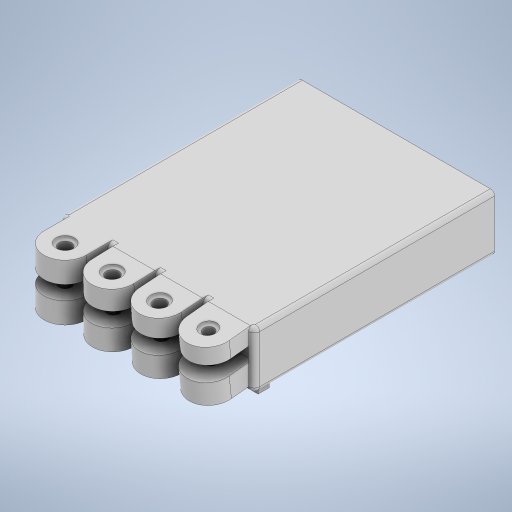
# Autodesk Inventor part: baze
Saved by Autodesk Inventor 2024 (Build 280153000, 153)
## iProperties
Created: 2023-12-07
Part Number: baze
Material: Типовые
Document SubType Name: Modeling
Designer: stefa
Density: 1 g/cm^3
Appearance: По умолчанию
Author: stefa
Autodesk Inventor part; units mm, degrees
ref_plane "YZ Plane" through (0, 0, 0) normal (1, 0, 0) x (0, 1, 0)
ref_plane "XZ Plane" through (0, 0, 0) normal (0, 1, 0) x (-1, 0, 0)
ref_plane "XY Plane" through (0, 0, 0) normal (0, 0, 1) x (1, 0, 0)
sketch "Эскиз1" plane through (0, 0, 0) normal (1, 0, 0) x (0, 1, 0)
  line L0 (0, 0) -> (20, 0)
  line L1 (20, 0) -> (20, -100)
  line L2 (20, -100) -> (0, -100)
  line L3 (0, -100) -> (0, 0)
  line L4 (12.5, 0) -> (12.5, -15)
  line L5 (12.5, -15) -> (7.5, -15)
  line L6 (7.5, -15) -> (7.5, 0)
  line L7 (7.5, 0) -> (12.5, 0)
  dimension "d0" = 20
  dimension "d1" = 100
  dimension "d2" = 15
  dimension "d3" = 5
  dimension "d4" = 7.5
  dimension "d5" = 7.5
  constraints: 16 end point, 4 parallel, 3 perpendicular, 1 horizontal, 1 point on line
  measures "d0" distance of L0.start L0.end
  measures "d1" distance of L0.end L1.end
  measures "d2" distance of L5.end L6.end
  measures "d3" distance of L4.end L5.end
  measures "d4" distance between parallel lines of L1 L4
  measures "d5" distance between parallel lines of L3 L6
extrude "Выдавливание1" add sketch "Эскиз1" along normal blind 15 contours L0 L6 L5 L4 L1 L2 L3
sketch "Эскиз2" plane through (15, 0, 0) normal (1, 0, 0) x (0, 0, -1)
  line L0 (0, 0) -> (100, 0) projected
  line L1 (100, 20) -> (0, 20) projected
  line L2 (100, 0) -> (15, 0)
  line L3 (15, 0) -> (15, 20)
  line L4 (15, 20) -> (100, 20)
  line L5 (100, 20) -> (100, 0)
  dimension "d8" = 85
  constraints: 8 end point, 2 parallel, 1 horizontal, 1 perpendicular, 1 point on line
  measures "d8" distance of L3.end L4.end
extrude "Выдавливание2" add sketch "Эскиз2" along normal blind 2
sketch "Эскиз3" plane through (17, 0, 0) normal (1, 0, 0) x (0, 0, -1)
  line L0 (100, 0) -> (100, 20)
  line L1 (0, 0) -> (100, 0)
  line L2 (100, 0) -> (100, 20)
  line L3 (100, 20) -> (0, 20)
  line L4 (0, 20) -> (0, 0)
  line L5 (0, 12.503049) -> (15, 13.02686)
  line L6 (15, 13.02686) -> (15.174604, 8.02686)
  line L7 (15.174604, 8.02686) -> (0, 7.496951)
  line L8 (0, 12.5) -> (15, 12.5)
  line L9 (0, 19.476188) -> (15, 20)
  line L10 (0, 0) -> (15, 0.523812)
  line L11 (15, 20) -> (15, 0)
  line L12 (15, 20) -> (15, 13.02686)
  line L13 (15.174604, 8.02686) -> (15, 0.523812)
  line L14 (15, 0) -> (15, 0.523812)
  line L15 (0, 19.476188) -> (0.243211, 12.511542)
  line L16 (0, 7.496951) -> (0.26148, 0.009131)
  dimension "d11" = 88
  dimension "d12" = 90
  dimension "d13" = 88
  dimension "d14" = 15
  dimension "d15" = 5
  dimension "d16" = 7.49695
  dimension "d17" = 7.49695
  dimension "d18" = 2
  dimension "d35" = 2
  dimension "d36" = 178
  dimension "d50" = 2
  dimension "d51" = 2
  constraints: 28 end point, 7 point on line, 2 parallel, 2 perpendicular, 1 collinear, 1 horizontal
  measures "d11" angle of L5 L4
  measures "d12" angle of L6 L7
  measures "d13" angle of L4 L7
  measures "d14" horizontal distance of L5.start L5.end
  measures "d15" vertical distance of L5.end L6.end
  measures "d16" distance of L3.end L5.start
  measures "d17" distance of L1.start L7.end
  measures "d18" angle of L8 L5
  measures "d35" angle of L3 L9
  measures "d36" angle of L1 L10
  measures "d50" angle of L15 L4
  measures "d51" angle of L16 L4
extrude "Выдавливание3" add sketch "Эскиз3" along normal blind 15 contours L1 L11 L13 L6 L3 L0 | L11 L5 L15 L9 | L10 L16 L7 L11 | L11 L7 L13
sketch "Эскиз4" plane through (32, 0, 0) normal (1, 0, 0) x (0, 0, -1)
  line L0 (15, 0) -> (15, 7.5) projected
  line L1 (100, 20) -> (15, 20) projected
  line L2 (15, 0) -> (100, 0)
  line L3 (100, 0) -> (100, 20)
  line L4 (100, 20) -> (15, 20)
  line L5 (15, 20) -> (15, 0)
  point P0 (0, 0)
  point P1 (0, 20)
  point P2 (15, 20)
  constraints: 8 end point, 2 parallel, 1 horizontal, 1 perpendicular
extrude "Выдавливание4" add sketch "Эскиз4" along normal blind 2
sketch "Эскиз5" plane through (34, 0, 0) normal (1, 0, 0) x (0, 0, -1)
  line L0 (15, 20) -> (0, 20)
  line L1 (100, 0) -> (100, 20)
  line L2 (0, 20) -> (100, 20)
  line L3 (100, 20) -> (100, 0)
  line L4 (100, 0) -> (0, 0)
  line L5 (0, 0) -> (0, 20)
  line L6 (0, 12.5) -> (15, 13.548902)
  line L7 (15, 13.548902) -> (15.347933, 8.573232)
  line L8 (15.347933, 8.573232) -> (0, 7.5)
  line L9 (15, 12.5) -> (15, 20)
  line L10 (0, 18.951098) -> (15, 20)
  line L11 (0, 0) -> (15, 1.048902)
  line L12 (15, 0) -> (15, 7.5)
  line L13 (15, 1.048902) -> (15, 0)
  line L14 (15, 0) -> (15, 20)
  line L15 (0, 18.951098) -> (0.44891, 12.531391)
  line L16 (0, 7.5) -> (0.521899, 0.036495)
  point P0 (0, 0)
  dimension "d23" = 90
  dimension "d24" = 90
  dimension "d25" = 86
  dimension "d26" = 86
  dimension "d27" = 5
  dimension "d28" = 7.5
  dimension "d29" = 7.5
  dimension "d30" = 15
  dimension "d31" = 86
  dimension "d32" = 4
  dimension "d52" = 4
  dimension "d53" = 4
  constraints: 26 end point, 5 point on line, 2 collinear, 2 parallel, 2 perpendicular, 1 horizontal
  measures "d23" angle of L7 L6
  measures "d24" angle of L7 L8
  measures "d25" angle of L6 L5
  measures "d26" angle of L8 L5
  measures "d27" distance of L8.end L6.start
  measures "d28" distance of L6.start L0.end
  measures "d29" distance of point (0, 0) L8.end
  measures "d30" horizontal distance of L6.start L6.end
  measures "d31" angle of L10 L5
  measures "d32" angle of L4 L11
  measures "d52" angle of L15 L5
  measures "d53" angle of L16 L5
extrude "Выдавливание5" add sketch "Эскиз5" along normal blind 15 contours L2 L1 L4 L12 L14 L8 L7 L9 | L9 L6 L15 L10 | L14 L12 L11 L16 L8
sketch "Эскиз6" plane through (49, 0, 0) normal (1, 0, 0) x (0, 0, -1)
  line L0 (100, 0) -> (100, 20)
  line L1 (15, 13.02686) -> (15, 20)
  line L2 (100, 0) -> (15, 0)
  line L3 (15, 0) -> (15, 20)
  line L4 (15, 20) -> (100, 20)
  line L5 (100, 20) -> (100, 0)
  point P0 (0, 0)
  constraints: 8 end point, 2 parallel, 1 horizontal, 1 perpendicular
extrude "Выдавливание6" add sketch "Эскиз6" along normal blind 2
sketch "Эскиз7" plane through (51, 0, 0) normal (1, 0, 0) x (0, 0, -1)
  line L0 (15, 20) -> (0, 20)
  line L1 (0, 0) -> (100, 0)
  line L2 (0, 20) -> (100, 20)
  line L3 (100, 20) -> (100, 0)
  line L4 (100, 0) -> (0, 0)
  line L5 (0, 0) -> (0, 20)
  line L6 (0, 12.5) -> (15, 14.076564)
  line L7 (15, 14.076564) -> (15.519779, 9.131195)
  line L8 (15.519779, 9.131195) -> (0, 7.5)
  line L9 (0, 18.423436) -> (15, 20)
  line L10 (0, 0) -> (15.064586, 1.583352)
  line L11 (15, 20) -> (15, 14.076564)
  line L12 (15.519779, 9.131195) -> (15.064586, 1.583352)
  line L13 (15.064586, 1.583352) -> (15, 0)
  line L14 (0, 18.423436) -> (0.615776, 12.564721)
  line L15 (0, 7.5) -> (0.779669, 0.081946)
  dimension "d39" = 90
  dimension "d40" = 90
  dimension "d41" = 84
  dimension "d42" = 5
  dimension "d43" = 7.5
  dimension "d44" = 7.5
  dimension "d45" = 15
  dimension "d46" = 84
  dimension "d47" = 6
  dimension "d54" = 6
  dimension "d55" = 6
  constraints: 28 end point, 7 point on line, 2 parallel, 2 perpendicular, 1 horizontal
  measures "d39" angle of L7 L6
  measures "d40" angle of L7 L8
  measures "d41" angle of L6 L5
  measures "d42" distance of L8.end L6.start
  measures "d43" distance of L1.start L8.end
  measures "d44" distance of L6.start L0.end
  measures "d45" horizontal distance of L6.end L6.start
  measures "d46" angle of L9 L5
  measures "d47" angle of L1 L10
  measures "d54" angle of L14 L5
  measures "d55" angle of L5 L15
extrude "Выдавливание7" add sketch "Эскиз7" along normal blind 15 contours L11 L6 L14 L9 | L2 L3 L1 L13 L12 L7 L11 | L12 L10 L15 L8
sketch "Эскиз8" plane through (0, 20, 0) normal (0, 1, 0) x (1, 0, 0)
  line L0 (0, 0) -> (15, 0) projected
  line L1 (0, 15) -> (15, 15) projected
  line L2 (0, 0) -> (15, 0)
  line L3 (15, 0) -> (15, 15)
  line L4 (15, 15) -> (0, 15)
  line L5 (0, 15) -> (0, 0)
  circle A0 centre (7.5, 7.5) radius 2.25
  dimension "d56" = 4.5
  constraints: 8 end point, 2 parallel, 1 centre point, 1 horizontal, 1 perpendicular
  measures "d56" diameter of A0
extrude "Выдавливание8" cut sketch "Эскиз8" against normal through all contours A0
sketch "Эскиз9" plane through (17, 19.476188, 0) normal (0, 0.9993908, 0.0348995) x (1, 0, 0)
  line L0 (0, -0.418069) -> (15, -0.418069)
  line L1 (0, 15.009143) -> (15, 15.009143)
  line L2 (0, -0.418069) -> (15, -0.418069)
  line L3 (15, -0.418069) -> (15, 15.009143)
  line L4 (15, 15.009143) -> (0, 15.009143)
  line L5 (0, 15.009143) -> (0, -0.418069)
  circle A0 centre (7.5, 7.295537) radius 2.25
  point P0 (-17, -0.679709)
  dimension "d59" = 4.5
  constraints: 8 end point, 2 parallel, 1 centre point, 1 horizontal, 1 perpendicular
  measures "d59" diameter of A0
extrude "Выдавливание9" cut sketch "Эскиз9" against normal through all contours A0
sketch "Эскиз10" plane through (34, 18.951098, 0) normal (0, 0.9975641, 0.0697565) x (1, 0, 0)
  line L0 (0, 14.23784) -> (0, -0.798788)
  line L1 (0, 15.036628) -> (15, 15.036628)
  line L2 (0, -0.798788) -> (15, -0.798788)
  line L3 (15, -0.798788) -> (15, 15.036628)
  line L4 (15, 15.036628) -> (0, 15.036628)
  line L5 (0, 15.036628) -> (0, -0.798788)
  circle A0 centre (7.5, 7.11892) radius 2.25
  point P0 (-34, -1.321962)
  dimension "d62" = 4.5
  constraints: 8 end point, 2 parallel, 1 centre point, 1 horizontal, 1 perpendicular
  measures "d62" diameter of A0
extrude "Выдавливание10" cut sketch "Эскиз10" against normal through all contours A0
sketch "Эскиз11" plane through (51, 18.423436, 0) normal (0, 0.9945219, 0.1045285) x (1, 0, 0)
  line L0 (0, 15.082624) -> (0, 0)
  line L1 (15, 99.616985) -> (15, 15.082624)
  line L2 (0, 0) -> (15, 0)
  line L3 (15, 0) -> (15, 15.082624)
  line L4 (15, 15.082624) -> (0, 15.082624)
  line L5 (0, 15.082624) -> (0, 0)
  circle A0 centre (7.5, 7.541312) radius 1.887312
  point P0 (-51, -1.925774)
  point P1 (0, -1.14181)
  constraints: 8 end point, 2 parallel, 1 centre point, 1 horizontal, 1 perpendicular
extrude "Выдавливание11" cut sketch "Эскиз11" against normal through all contours A0
sketch "Эскиз12" plane through (0, 0, -100) normal (0, -1, 0) x (1, 0, 0)
  point P0 (0, 100)
sketch "Эскиз13" plane through (0, 0, -100) normal (0, -1, 0) x (1, 0, 0)
  line L0 (52.25, 23.25) -> (64.75, 23.25)
  line L1 (64.75, 23.25) -> (64.75, 46.75)
  line L2 (64.75, 46.75) -> (52.25, 46.75)
  line L3 (52.25, 46.75) -> (52.25, 23.25)
  line L4 (52.25, 23.25) -> (64.75, 46.75) construction
  line L5 (64.75, 23.25) -> (52.25, 46.75) construction
  line L6 (35.25, 26.75) -> (47.75, 26.75)
  line L7 (47.75, 26.75) -> (47.75, 3.25)
  line L8 (47.75, 3.25) -> (35.25, 3.25)
  line L9 (35.25, 3.25) -> (35.25, 26.75)
  line L10 (35.25, 26.75) -> (47.75, 3.25) construction
  line L11 (47.75, 26.75) -> (35.25, 3.25) construction
  line L12 (18.25, 46.75) -> (30.75, 46.75)
  line L13 (30.75, 46.75) -> (30.75, 23.25)
  line L14 (30.75, 23.25) -> (18.25, 23.25)
  line L15 (18.25, 23.25) -> (18.25, 46.75)
  line L16 (18.25, 46.75) -> (30.75, 23.25) construction
  line L17 (30.75, 46.75) -> (18.25, 23.25) construction
  line L18 (1.25, 26.75) -> (13.75, 26.75)
  line L19 (13.75, 26.75) -> (13.75, 3.25)
  line L20 (13.75, 3.25) -> (1.25, 3.25)
  line L21 (1.25, 3.25) -> (1.25, 26.75)
  line L22 (1.25, 26.75) -> (13.75, 3.25) construction
  line L23 (13.75, 26.75) -> (1.25, 3.25) construction
  line L24 (66, 85) -> (66, 0) projected
  line L25 (0, 100) -> (0, 0) projected
  line L26 (51, 85) -> (66, 85) projected
  line L27 (15, 85) -> (51, 85) projected
  line L28 (0, 85) -> (15, 85) projected
  point P0 (58.5, 35)
  point P1 (41.5, 15)
  point P2 (24.5, 35)
  point P3 (7.5, 15)
  dimension "d68" = 12.5
  dimension "d69" = 7.5
  dimension "d70" = 17
  dimension "d71" = 17
  dimension "d72" = 17
  dimension "d73" = 7.5
  dimension "d74" = 12.5
  dimension "d75" = 12.5
  dimension "d76" = 12.5
  dimension "d77" = 23.5
  dimension "d78" = 23.5
  dimension "d79" = 23.5
  dimension "d80" = 23.5
  dimension "d81" = 50
  dimension "d82" = 70
  dimension "d83" = 50
  dimension "d84" = 70
  constraints: 48 end point, 8 midpoint, 8 parallel, 4 horizontal, 4 perpendicular
  measures "d68" distance of L0.start L0.end
  measures "d69" distance from line of L24 point (58.5, 35)
  measures "d70" horizontal distance of point (58.5, 35) point (41.5, 15)
  measures "d71" horizontal distance of point (24.5, 35) point (41.5, 15)
  measures "d72" horizontal distance of point (7.5, 15) point (24.5, 35)
  measures "d73" distance from line of L25 point (7.5, 15)
  measures "d74" distance of L13.end L14.end
  measures "d75" distance of L19.end L20.end
  measures "d76" distance of L7.end L8.end
  measures "d77" distance of L2.end L0.start
  measures "d78" distance of L8.end L6.start
  measures "d79" distance of L12.end L13.end
  measures "d80" distance of L18.end L19.end
  measures "d81" distance from line of L26 point (58.5, 35)
  measures "d82" distance from line of L27 point (41.5, 15)
  measures "d83" distance from line of L27 point (24.5, 35)
  measures "d84" distance from line of L28 point (7.5, 15)
extrude "Выдавливание12" cut sketch "Эскиз13" against normal blind 17
sketch "Эскиз14" plane through (66, 0, 0) normal (1, 0, 0) x (0, 0, -1)
  line L0 (100, 0) -> (100, 20)
  line L1 (100, 0) -> (14.318548, 0)
  line L2 (14.318548, 0) -> (14.318548, 20)
  line L3 (14.318548, 20) -> (100, 20)
  line L4 (100, 20) -> (100, 0)
  point P0 (0, 0)
  constraints: 8 end point, 2 parallel, 1 horizontal, 1 perpendicular
extrude "Выдавливание13" add sketch "Эскиз14" along normal blind 2
sketch "Эскиз15" plane through (0, 0, 0) normal (-1, 0, 0) x (0, 0, 1)
  line L0 (0, 0) -> (-100, 0) projected
  line L1 (-100, 0) -> (-15, 0)
  line L2 (-15, 0) -> (-15, 20)
  line L3 (-15, 20) -> (-100, 20)
  line L4 (-100, 20) -> (-100, 0)
  constraints: 8 end point, 2 parallel, 1 horizontal, 1 perpendicular
extrude "Выдавливание14" add sketch "Эскиз15" along normal blind 2
sketch "Эскиз16" plane through (0, 0, -15) normal (0, -1, 0) x (1, 0, 0)
  line L0 (63.5, -5.25) -> (53.5, -5.25)
  line L1 (53.5, -5.25) -> (53.5, -9.25)
  line L2 (53.5, -9.25) -> (63.5, -9.25)
  line L3 (63.5, -9.25) -> (63.5, -5.25)
  line L4 (46.5, -5.25) -> (36.5, -5.25)
  line L5 (36.5, -5.25) -> (36.5, -9.25)
  line L6 (36.5, -9.25) -> (46.5, -9.25)
  line L7 (46.5, -9.25) -> (46.5, -5.25)
  line L8 (29.5, -5.25) -> (19.5, -5.25)
  line L9 (19.5, -5.25) -> (19.5, -9.25)
  line L10 (19.5, -9.25) -> (29.5, -9.25)
  line L11 (29.5, -9.25) -> (29.5, -5.25)
  line L12 (12.5, -5.25) -> (2.5, -5.25)
  line L13 (2.5, -5.25) -> (2.5, -9.25)
  line L14 (2.5, -9.25) -> (12.5, -9.25)
  line L15 (12.5, -9.25) -> (12.5, -5.25)
  line L16 (52.25, -38.25) -> (64.75, -38.25)
  line L17 (68, 0.681452) -> (68, -85)
  line L18 (-2, -85) -> (-2, 0)
  line L19 (51, 0) -> (66, 0)
  line L20 (15, 0) -> (51, 0)
  point P0 (0, 15)
  point P1 (58.5, -5.25)
  point P2 (41.5, -5.25)
  point P3 (24.5, -5.25)
  point P4 (7.5, -5.25)
  dimension "d91" = 10
  dimension "d92" = 10
  dimension "d93" = 10
  dimension "d94" = 10
  dimension "d95" = 4
  dimension "d96" = 4
  dimension "d97" = 4
  dimension "d98" = 0
  dimension "d99" = 29
  dimension "d100" = 9.5
  dimension "d101" = 17
  dimension "d102" = 17
  dimension "d103" = 17
  dimension "d104" = 9.5
  dimension "d138" = 5.25
  dimension "d139" = 5.25
  constraints: 32 end point, 8 parallel, 4 horizontal, 4 midpoint, 4 perpendicular, 3 point on line
  measures "d91" distance of L9.end L10.end
  measures "d92" distance of L13.end L14.end
  measures "d93" distance of L5.end L6.end
  measures "d94" distance of L1.end L2.end
  measures "d95" distance of L0.end L1.end
  measures "d96" distance of L8.end L9.end
  measures "d97" distance of L12.end L13.end
  measures "d98" distance between parallel lines of L8 L12
  measures "d99" distance between parallel lines of L16 L2
  measures "d100" distance from line of point (58.5, -5.25) L17
  measures "d101" distance of point (58.5, -5.25) point (41.5, -5.25)
  measures "d102" distance of point (41.5, -5.25) point (24.5, -5.25)
  measures "d103" distance of point (24.5, -5.25) point (7.5, -5.25)
  measures "d104" distance from line of L18 point (7.5, -5.25)
  measures "d138" distance between parallel lines of L19 L0
  measures "d139" distance between parallel lines of L20 L8
extrude "Выдавливание15" add sketch "Эскиз16" along normal blind 5
sketch "Эскиз17" plane through (63.5, 0, -24.25) normal (0, 0, -1) x (-1, 0, 0)
  line L0 (2.5, -3.384771) -> (7.5, -3.384771)
  line L1 (7.5, -3.384771) -> (7.5, -1.384771)
  line L2 (7.5, -1.384771) -> (2.5, -1.384771)
  line L3 (2.5, -1.384771) -> (2.5, -3.384771)
  line L4 (19.5, -3.384771) -> (24.5, -3.384771)
  line L5 (24.5, -3.384771) -> (24.5, -1.384771)
  line L6 (24.5, -1.384771) -> (19.5, -1.384771)
  line L7 (19.5, -1.384771) -> (19.5, -3.384771)
  line L8 (36.5, -3.384771) -> (41.5, -3.384771)
  line L9 (41.5, -3.384771) -> (41.5, -1.384771)
  line L10 (41.5, -1.384771) -> (36.5, -1.384771)
  line L11 (36.5, -1.384771) -> (36.5, -3.384771)
  line L12 (53.5, -3.384771) -> (58.5, -3.384771)
  line L13 (58.5, -3.384771) -> (58.5, -1.384771)
  line L14 (58.5, -1.384771) -> (53.5, -1.384771)
  line L15 (53.5, -1.384771) -> (53.5, -3.384771)
  line L16 (0, 0) -> (0, -5)
  line L17 (10, 0) -> (10, -5)
  line L18 (17, 0) -> (17, -5)
  line L19 (34, 0) -> (34, -5)
  line L20 (51, 0) -> (51, -5)
  point P0 (63.5, 0)
  point P1 (51, -2.5)
  dimension "d107" = 2
  dimension "d108" = 5
  dimension "d109" = 5
  dimension "d110" = 5
  dimension "d111" = 5
  dimension "d112" = 2.5
  dimension "d113" = 2.5
  dimension "d114" = 2.5
  dimension "d115" = 2.5
  dimension "d116" = 2.5
  constraints: 32 end point, 8 parallel, 6 point on line, 4 horizontal, 4 perpendicular, 1 midpoint
  measures "d107" distance of L0.end L1.end
  measures "d108" distance of L0.start L0.end
  measures "d109" distance of L4.start L4.end
  measures "d110" distance of L8.start L8.end
  measures "d111" distance of L12.start L12.end
  measures "d112" distance between parallel lines of L16 L3
  measures "d113" distance between parallel lines of L17 L1
  measures "d114" distance between parallel lines of L18 L7
  measures "d115" distance between parallel lines of L19 L11
  measures "d116" distance from line of point (51, -2.5) L15
extrude "Выдавливание16" cut sketch "Эскиз17" against normal up to surface (4 mm away)
fillet "Сопряжение1" radius 1.5 10 edges at (68, 20, -57.1593) (67, 20, -14.3185) (-1, 20, -15) (-2, 20, -57.5) (68, 0, -57.1593) (67, 0, -14.3185) (58.5, 0, -15) (33, 0, -15) (-1, 0, -15) (-2, 0, -57.5)
fillet "Сопряжение2" radius 2 3 edges at (50, 20, -15) (16, 20, -15) (33, 20, -15)
fillet "Сопряжение3" radius 2 6 edges at (-1.5607, 19.5607, -15.4393) (-1.5607, 0.4393, -15.4393) (-2, 10, -15) (67.5607, 0.4393, -14.7579) (67.5607, 19.5607, -14.7579) (68, 10, -14.3185)
fillet "Сопряжение4" radius 7.5 16 edges at (0, 16.25, 0) (15, 16.25, 0) (17, 15.9939, -0.1216) (32, 15.9939, -0.1216) (34, 15.7412, -0.2245) (49, 15.7412, -0.2245) (66, 15.4941, -0.3079) (51, 15.4941, -0.3079) (66, 3.791, -0.3898) (51, 3.791, -0.3898) (49, 3.7682, -0.2609) (34, 3.7682, -0.2609) (32, 3.753, -0.1307) (15, 3.75, 0) (0, 3.75, 0) (17, 3.753, -0.1307)
fillet "Сопряжение5" radius 1 10 edges at (58.5, -3.3848, -24.25) (61, -2.3848, -24.25) (58.5, -1.3848, -24.25) (56, -2.3848, -24.25) (61, -2.3848, -20.25) (58.5, -3.3848, -20.25) (58.5, -1.3848, -20.25) (56, -2.3848, -20.25) (61, -1.3848, -22.25) (56, -1.3848, -22.25)
fillet "Сопряжение6" radius 1 10 edges at (44, -2.3848, -24.25) (44, -1.3848, -22.25) (39, -1.3848, -22.25) (41.5, -1.3848, -24.25) (39, -2.3848, -24.25) (41.5, -3.3848, -24.25) (41.5, -3.3848, -20.25) (44, -2.3848, -20.25) (41.5, -1.3848, -20.25) (39, -2.3848, -20.25)
fillet "Сопряжение7" radius 1 10 edges at (27, -1.3848, -22.25) (22, -1.3848, -22.25) (24.5, -1.3848, -20.25) (24.5, -1.3848, -24.25) (27, -2.3848, -24.25) (27, -2.3848, -20.25) (22, -2.3848, -24.25) (22, -2.3848, -20.25) (24.5, -3.3848, -24.25) (24.5, -3.3848, -20.25)
fillet "Сопряжение8" radius 1 10 edges at (7.5, -3.3848, -24.25) (7.5, -3.3848, -20.25) (10, -2.3848, -24.25) (10, -2.3848, -20.25) (10, -1.3848, -22.25) (5, -1.3848, -22.25) (5, -2.3848, -24.25) (5, -2.3848, -20.25) (7.5, -1.3848, -24.25) (7.5, -1.3848, -20.25)
sketch "Эскиз18" plane through (53.5, 0, -24.25) normal (0, -1, 0) x (1, 0, 0)
  line L0 (-1.25, -32.5) -> (11.25, -32.5) projected
  line L1 (13, -75.75) -> (-54, -75.75) projected
  line L2 (8, -32.5) -> (2, -32.5)
  line L3 (2, -32.5) -> (2, -75.75)
  line L4 (2, -75.75) -> (8, -75.75)
  line L5 (8, -75.75) -> (8, -32.5)
  line L6 (-18.25, -52.5) -> (-5.75, -52.5) projected
  line L7 (-9, -52.5) -> (-15, -52.5)
  line L8 (-15, -52.5) -> (-15, -75.75)
  line L9 (-15, -75.75) -> (-9, -75.75)
  line L10 (-9, -75.75) -> (-9, -52.5)
  line L11 (-26, -32.5) -> (-32, -32.5)
  line L12 (-32, -32.5) -> (-32, -75.75)
  line L13 (-32, -75.75) -> (-26, -75.75)
  line L14 (-26, -75.75) -> (-26, -32.5)
  line L15 (-52.25, -49) -> (-39.75, -49) projected
  line L16 (-43, -49) -> (-49, -49)
  line L17 (-49, -49) -> (-49, -75.75)
  line L18 (-49, -75.75) -> (-43, -75.75)
  line L19 (-43, -75.75) -> (-43, -49)
  line L20 (11.25, -29) -> (11.25, -52.5) projected
  line L21 (-1.25, -52.5) -> (-1.25, -29) projected
  line L22 (-5.75, -49) -> (-5.75, -72.5) projected
  line L23 (-22.75, -29) -> (-22.75, -52.5) projected
  line L24 (-39.75, -49) -> (-39.75, -72.5) projected
  point P0 (-53.5, 24.25)
  point P1 (-43, -75.75)
  point P2 (-49, -75.75)
  point P3 (-32, -75.75)
  point P4 (-26, -75.75)
  point P5 (-9, -75.75)
  point P6 (-15, -75.75)
  point P7 (2, -32.5)
  dimension "d127" = 6
  dimension "d128" = 6
  dimension "d129" = 6
  dimension "d130" = 6
  dimension "d131" = 3.25
  dimension "d132" = 3.25
  dimension "d133" = 3.25
  dimension "d134" = 3.25
  dimension "d135" = 3.25
  constraints: 32 end point, 8 parallel, 8 point on line, 4 horizontal, 4 perpendicular
  measures "d127" distance between parallel lines of L12 L14
  measures "d128" distance between parallel lines of L17 L19
  measures "d129" distance between parallel lines of L8 L10
  measures "d130" distance between parallel lines of L5 L3
  measures "d131" distance between parallel lines of L20 L5
  measures "d132" distance between parallel lines of L21 L3
  measures "d133" distance between parallel lines of L22 L10
  measures "d134" distance between parallel lines of L23 L14
  measures "d135" distance between parallel lines of L24 L19
extrude "Выдавливание17" cut sketch "Эскиз18" against normal blind 15
fillet "Сопряжение9" radius 1 8 edges at (5.25, 20, -7.5) (22.25, 19.7308, -7.2911) (39.25, 19.4477, -7.1016) (56.6127, 19.2117, -7.5) (56.6127, 0.9896, -9.4152) (39.25, 0.5888, -8.4203) (22.25, 0.2783, -7.9704) (5.25, 0, -7.5) inverted yes
equation "\"d4\" = d5"
equation "\"d16\" = d17"
equation "\"d28\" = d29"
equation "\"d43\" = d44"
equation "\"d112\" = d113"
equation "\"d131\" = d132"
